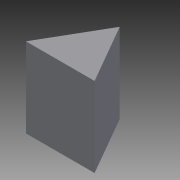
# Autodesk Inventor part: 129_4
Saved by Autodesk Inventor 2014 (Build 180170000, 170)
## iProperties
Created: 2017-04-22
Part Number: 129_4
Material: Generic
Document SubType Name: Modeling
Designer: Andy
Density: 1 g/cm^3
Appearance: Default
Author: Andy
Autodesk Inventor part; units mm, degrees
ref_plane "YZ Plane" through (0, 0, 0) normal (1, 0, 0) x (0, 1, 0)
ref_plane "XZ Plane" through (0, 0, 0) normal (0, 1, 0) x (-1, 0, 0)
ref_plane "XY Plane" through (0, 0, 0) normal (0, 0, 1) x (1, 0, 0)
sketch "Sketch1" plane through (0, 0, 0) normal (0, 1, 0) x (-1, 0, 0)
  line L0 (0, -4.9738) -> (-4.3074, 2.4869)
  line L1 (-4.3074, 2.4869) -> (4.3074, 2.4869)
  line L2 (4.3074, 2.4869) -> (0, -4.9738)
  point P0 (0, 0)
  point P1 (0, 0)
  constraints: 6 end point, 1 coincident, 7 other
extrude "Extrusion1" add sketch "Sketch1" along normal blind 10
body "Solid1"
